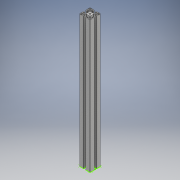
# Autodesk Inventor part: Perfil de Aluminio
Saved by Autodesk Inventor 2018.3 (Build 223284000, 284)
## iProperties
Created: 2020-12-03
Part Number: Perfil de Aluminio
Material: Aluminio 6061
Document SubType Name: Modeling
Designer: SERGIO ROMO
Density: 2.7 g/cm^3
Appearance: Aluminio fundido
Author: SERGIO ROMO
Revision Number: ANY
Autodesk Inventor part; units mm, degrees
ref_plane "YZ Plane" through (0, 0, 0) normal (1, 0, 0) x (0, 1, 0)
ref_plane "XZ Plane" through (0, 0, 0) normal (0, 1, 0) x (-1, 0, 0)
ref_plane "XY Plane" through (0, 0, 0) normal (0, 0, 1) x (1, 0, 0)
sketch "Boceto1" plane through (0, 0, 0) normal (0, 0, 1) x (1, 0, 0)
  line L0 (1.5, 20) -> (15.2768, 20) projected
  line L1 (15.2768, 20) -> (1.5, 20)
  line L2 (8, 12.6183) -> (8, 17.77) projected
  line L3 (8, 17.77) -> (8, 12.6183)
  line L4 (1.5, 12.6183) -> (1.5, 17) projected
  line L5 (2.23, 12) -> (7.3817, 12) projected
  line L6 (7.3817, 18.5) -> (3, 18.5) projected
  line L7 (7.3817, 18.5) -> (3, 18.5)
  arc A0 (3, 18.5) -> (1.9393, 18.0607) centre (3, 17) ccw
  arc A1 (8, 17.77) -> (7.3817, 18.5) centre (7.2949, 17.7996) ccw
  arc A2 (7.8053, 12.1947) -> (8, 12.6183) centre (7.3305, 12.6695) ccw
  line L8 (16, 19.2235) -> (16, 16.1235) projected
  line L9 (16, 19.2235) -> (16, 16.1235)
  circle A3 centre (20, 0) radius 3.4 projected
  arc A4 (1.5, 20) -> (0, 18.5) centre (1.5, 18.5) ccw projected
  arc A5 (1.5, 20) -> (0.4393, 19.5607) centre (1.5, 18.5) ccw
  line L10 (15.4384, 15.5) -> (13.3245, 15.5) projected
  line L11 (15.4384, 15.5) -> (13.3245, 15.5)
  line L12 (13, 15.7733) -> (13, 18.5) projected
  arc A6 (13, 18.5) -> (10, 15.5) centre (13, 15.5) ccw projected
  line L13 (13, 15.7733) -> (13, 18.5)
  line L14 (10, 13.2043) -> (10, 15.5) projected
  line L15 (10, 15.5) -> (10, 13.2043)
  arc A7 (16, 19.2235) -> (15.2768, 20) centre (15.0156, 19.0317) ccw
  arc A8 (15.4384, 15.5) -> (16, 16.1235) centre (15.3104, 16.1799) ccw
  arc A9 (13, 18.5) -> (10, 15.5) centre (13, 15.5) ccw
  line L16 (24, 7.75) -> (16, 7.75) projected
  line L17 (10.8789, 10.9836) -> (13.3701, 8.4924) projected
  line L18 (10.8789, 10.9836) -> (13.3701, 8.4924)
  arc A10 (10, 13.2043) -> (10.8789, 10.9836) centre (13.2448, 13.2043) ccw
  arc A11 (13.3701, 8.4924) -> (16, 7.75) centre (15.5379, 11.1424) ccw
  line L19 (7.3817, 12) -> (7.2793, 12)
  line L20 (2.3351, 12) -> (2.23, 12)
  arc A12 (13, 15.7733) -> (13.3245, 15.5) centre (13.4072, 15.9275) ccw
  line L21 (0, 18.5) -> (0, 4.7232)
  line L22 (7.3817, 12) -> (2.23, 12)
  line L23 (1.5, 12.6183) -> (1.5, 17)
  arc A13 (1.9393, 18.0607) -> (1.5, 17) centre (3, 17) ccw
  arc A14 (1.5, 12.6183) -> (2.23, 12) centre (2.2004, 12.7051) ccw
  arc A15 (7.3817, 12) -> (7.8053, 12.1947) centre (7.3305, 12.6695) ccw
  line L24 (0.7765, 4) -> (3.8765, 4)
  arc A16 (0.4393, 19.5607) -> (0, 18.5) centre (1.5, 18.5) ccw
  line L25 (4.5, 4.5616) -> (4.5, 6.6755)
  line L26 (4.2267, 7) -> (1.5, 7)
  line L27 (4.5, 10) -> (6.7957, 10)
  arc A17 (0, 4.7232) -> (0.7765, 4) centre (0.9683, 4.9844) ccw
  arc A18 (3.8765, 4) -> (4.5, 4.5616) centre (3.8201, 4.6896) ccw
  arc A19 (4.5, 10) -> (1.5, 7) centre (4.5, 7) ccw
  line L28 (12.25, 4) -> (12.25, 0)
  line L29 (9.0164, 9.1211) -> (11.5076, 6.6299)
  arc A20 (9.0164, 9.1211) -> (6.7957, 10) centre (6.7957, 6.7552) ccw
  arc A21 (12.25, 4) -> (11.5076, 6.6299) centre (8.8576, 4.4621) ccw
  arc A22 (4.5, 6.6755) -> (4.2267, 7) centre (4.0725, 6.5928) ccw
  line L30 (1.5, -20) -> (15.2768, -20)
  line L31 (15.2768, -20) -> (1.5, -20)
  line L32 (8, -12.6183) -> (8, -17.77)
  line L33 (8, -17.77) -> (8, -12.6183)
  line L34 (1.5, -12.6183) -> (1.5, -17)
  line L35 (2.23, -12) -> (7.3817, -12)
  line L36 (7.3817, -18.5) -> (3, -18.5)
  line L37 (7.3817, -18.5) -> (3, -18.5)
  arc A23 (1.9393, -18.0607) -> (3, -18.5) centre (3, -17) ccw
  arc A24 (7.3817, -18.5) -> (8, -17.77) centre (7.2949, -17.7996) ccw
  arc A25 (8, -12.6183) -> (7.8053, -12.1947) centre (7.3305, -12.6695) ccw
  line L38 (16, -19.2235) -> (16, -16.1235)
  arc A26 (0, -18.5) -> (1.5, -20) centre (1.5, -18.5) ccw
  arc A27 (0.4393, -19.5607) -> (1.5, -20) centre (1.5, -18.5) ccw
  line L39 (15.4384, -15.5) -> (13.3245, -15.5)
  line L40 (13, -15.7733) -> (13, -18.5)
  arc A28 (10, -15.5) -> (13, -18.5) centre (13, -15.5) ccw
  line L41 (13, -15.7733) -> (13, -18.5)
  line L42 (10, -13.2043) -> (10, -15.5)
  line L43 (10, -15.5) -> (10, -13.2043)
  arc A29 (15.2768, -20) -> (16, -19.2235) centre (15.0156, -19.0317) ccw
  arc A30 (16, -16.1235) -> (15.4384, -15.5) centre (15.3104, -16.1799) ccw
  arc A31 (10, -15.5) -> (13, -18.5) centre (13, -15.5) ccw
  line L44 (24, -7.75) -> (16, -7.75)
  line L45 (10.8789, -10.9836) -> (13.3701, -8.4924)
  line L46 (10.8789, -10.9836) -> (13.3701, -8.4924)
  arc A32 (10.8789, -10.9836) -> (10, -13.2043) centre (13.2448, -13.2043) ccw
  arc A33 (16, -7.75) -> (13.3701, -8.4924) centre (15.5379, -11.1424) ccw
  line L47 (7.3817, -12) -> (7.2793, -12)
  line L48 (2.3351, -12) -> (2.23, -12)
  arc A34 (13.3245, -15.5) -> (13, -15.7733) centre (13.4072, -15.9275) ccw
  arc A35 (0, -18.5) -> (0.4393, -19.5607) centre (1.5, -18.5) ccw
  line L49 (0, -18.5) -> (0, -4.7232)
  arc A36 (0.7765, -4) -> (0, -4.7232) centre (0.9683, -4.9844) ccw
  line L50 (0.7765, -4) -> (3.8765, -4)
  arc A37 (4.5, -4.5616) -> (3.8765, -4) centre (3.8201, -4.6896) ccw
  line L51 (4.5, -4.5616) -> (4.5, -6.6755)
  arc A38 (4.2267, -7) -> (4.5, -6.6755) centre (4.0725, -6.5928) ccw
  line L52 (4.2267, -7) -> (1.5, -7)
  arc A39 (1.5, -7) -> (4.5, -10) centre (4.5, -7) ccw
  line L53 (4.5, -10) -> (6.7957, -10)
  arc A40 (6.7957, -10) -> (9.0164, -9.1211) centre (6.7957, -6.7552) ccw
  line L54 (9.0164, -9.1211) -> (11.5076, -6.6299)
  arc A41 (11.5076, -6.6299) -> (12.25, -4) centre (8.8576, -4.4621) ccw
  line L55 (12.25, -4) -> (12.25, 0)
  arc A42 (7.8053, -12.1947) -> (7.3817, -12) centre (7.3305, -12.6695) ccw
  line L56 (7.3817, -12) -> (2.23, -12)
  arc A43 (2.23, -12) -> (1.5, -12.6183) centre (2.2004, -12.7051) ccw
  line L57 (1.5, -12.6183) -> (1.5, -17)
  arc A44 (1.5, -17) -> (1.9393, -18.0607) centre (3, -17) ccw
  line L58 (38.5, 20) -> (24.7232, 20)
  line L59 (24.7232, 20) -> (38.5, 20)
  line L60 (32, 12.6183) -> (32, 17.77)
  line L61 (32, 17.77) -> (32, 12.6183)
  line L62 (38.5, 12.6183) -> (38.5, 17)
  line L63 (37.77, 12) -> (32.6183, 12)
  line L64 (32.6183, 18.5) -> (37, 18.5)
  line L65 (32.6183, 18.5) -> (37, 18.5)
  arc A45 (38.0607, 18.0607) -> (37, 18.5) centre (37, 17) ccw
  arc A46 (32.6183, 18.5) -> (32, 17.77) centre (32.7051, 17.7996) ccw
  arc A47 (32, 12.6183) -> (32.1947, 12.1947) centre (32.6695, 12.6695) ccw
  line L66 (24, 19.2235) -> (24, 16.1235)
  line L67 (24, 19.2235) -> (24, 16.1235)
  arc A48 (40, 18.5) -> (38.5, 20) centre (38.5, 18.5) ccw
  arc A49 (39.5607, 19.5607) -> (38.5, 20) centre (38.5, 18.5) ccw
  line L68 (24.5616, 15.5) -> (26.6755, 15.5)
  line L69 (24.5616, 15.5) -> (26.6755, 15.5)
  line L70 (27, 15.7733) -> (27, 18.5)
  arc A50 (30, 15.5) -> (27, 18.5) centre (27, 15.5) ccw
  line L71 (27, 15.7733) -> (27, 18.5)
  line L72 (30, 13.2043) -> (30, 15.5)
  line L73 (30, 15.5) -> (30, 13.2043)
  arc A51 (24.7232, 20) -> (24, 19.2235) centre (24.9844, 19.0317) ccw
  arc A52 (24, 16.1235) -> (24.5616, 15.5) centre (24.6896, 16.1799) ccw
  arc A53 (30, 15.5) -> (27, 18.5) centre (27, 15.5) ccw
  line L74 (29.1211, 10.9836) -> (26.6299, 8.4924)
  line L75 (29.1211, 10.9836) -> (26.6299, 8.4924)
  arc A54 (29.1211, 10.9836) -> (30, 13.2043) centre (26.7552, 13.2043) ccw
  arc A55 (24, 7.75) -> (26.6299, 8.4924) centre (24.4621, 11.1424) ccw
  line L76 (32.6183, 12) -> (32.7207, 12)
  line L77 (37.6649, 12) -> (37.77, 12)
  arc A56 (26.6755, 15.5) -> (27, 15.7733) centre (26.5928, 15.9275) ccw
  arc A57 (40, 18.5) -> (39.5607, 19.5607) centre (38.5, 18.5) ccw
  line L78 (40, 18.5) -> (40, 4.7232)
  arc A58 (39.2235, 4) -> (40, 4.7232) centre (39.0317, 4.9844) ccw
  line L79 (39.2235, 4) -> (36.1235, 4)
  arc A59 (35.5, 4.5616) -> (36.1235, 4) centre (36.1799, 4.6896) ccw
  line L80 (35.5, 4.5616) -> (35.5, 6.6755)
  arc A60 (35.7733, 7) -> (35.5, 6.6755) centre (35.9275, 6.5928) ccw
  line L81 (35.7733, 7) -> (38.5, 7)
  arc A61 (38.5, 7) -> (35.5, 10) centre (35.5, 7) ccw
  line L82 (35.5, 10) -> (33.2043, 10)
  arc A62 (33.2043, 10) -> (30.9836, 9.1211) centre (33.2043, 6.7552) ccw
  line L83 (30.9836, 9.1211) -> (28.4924, 6.6299)
  arc A63 (28.4924, 6.6299) -> (27.75, 4) centre (31.1424, 4.4621) ccw
  line L84 (27.75, 4) -> (27.75, 0)
  arc A64 (32.1947, 12.1947) -> (32.6183, 12) centre (32.6695, 12.6695) ccw
  line L85 (32.6183, 12) -> (37.77, 12)
  arc A65 (37.77, 12) -> (38.5, 12.6183) centre (37.7996, 12.7051) ccw
  line L86 (38.5, 12.6183) -> (38.5, 17)
  arc A66 (38.5, 17) -> (38.0607, 18.0607) centre (37, 17) ccw
  arc A67 (38.0607, -18.0607) -> (38.5, -17) centre (37, -17) ccw
  arc A68 (37, -18.5) -> (38.0607, -18.0607) centre (37, -17) ccw
  arc A69 (38.5, -20) -> (39.5607, -19.5607) centre (38.5, -18.5) ccw
  arc A70 (39.5607, -19.5607) -> (40, -18.5) centre (38.5, -18.5) ccw
  arc A71 (38.5, -20) -> (40, -18.5) centre (38.5, -18.5) ccw
  line L87 (30, -13.2043) -> (30, -15.5)
  line L88 (29.1211, -10.9836) -> (26.6299, -8.4924)
  line L89 (29.1211, -10.9836) -> (26.6299, -8.4924)
  arc A72 (30, -13.2043) -> (29.1211, -10.9836) centre (26.7552, -13.2043) ccw
  line L90 (30, -15.5) -> (30, -13.2043)
  line L91 (38.5, -20) -> (24.7232, -20)
  line L92 (24.7232, -20) -> (38.5, -20)
  arc A73 (27, -15.7733) -> (26.6755, -15.5) centre (26.5928, -15.9275) ccw
  arc A74 (27, -18.5) -> (30, -15.5) centre (27, -15.5) ccw
  arc A75 (27, -18.5) -> (30, -15.5) centre (27, -15.5) ccw
  line L93 (27, -15.7733) -> (27, -18.5)
  line L94 (27, -15.7733) -> (27, -18.5)
  line L95 (27.75, -4) -> (27.75, 0)
  arc A76 (27.75, -4) -> (28.4924, -6.6299) centre (31.1424, -4.4621) ccw
  line L96 (30.9836, -9.1211) -> (28.4924, -6.6299)
  arc A77 (30.9836, -9.1211) -> (33.2043, -10) centre (33.2043, -6.7552) ccw
  arc A78 (36.1235, -4) -> (35.5, -4.5616) centre (36.1799, -4.6896) ccw
  line L97 (35.5, -4.5616) -> (35.5, -6.6755)
  arc A79 (35.5, -6.6755) -> (35.7733, -7) centre (35.9275, -6.5928) ccw
  line L98 (35.5, -10) -> (33.2043, -10)
  line L99 (39.2235, -4) -> (36.1235, -4)
  arc A80 (40, -4.7232) -> (39.2235, -4) centre (39.0317, -4.9844) ccw
  line L100 (35.7733, -7) -> (38.5, -7)
  arc A81 (35.5, -10) -> (38.5, -7) centre (35.5, -7) ccw
  line L101 (32, -12.6183) -> (32, -17.77)
  line L102 (32, -17.77) -> (32, -12.6183)
  line L103 (32.6183, -18.5) -> (37, -18.5)
  line L104 (32.6183, -18.5) -> (37, -18.5)
  arc A82 (32, -17.77) -> (32.6183, -18.5) centre (32.7051, -17.7996) ccw
  line L105 (40, -18.5) -> (40, -4.7232)
  line L106 (38.5, -12.6183) -> (38.5, -17)
  line L107 (38.5, -12.6183) -> (38.5, -17)
  arc A83 (38.5, -12.6183) -> (37.77, -12) centre (37.7996, -12.7051) ccw
  line L108 (37.6649, -12) -> (37.77, -12)
  line L109 (32.6183, -12) -> (37.77, -12)
  line L110 (37.77, -12) -> (32.6183, -12)
  line L111 (32.6183, -12) -> (32.7207, -12)
  arc A84 (32.6183, -12) -> (32.1947, -12.1947) centre (32.6695, -12.6695) ccw
  arc A85 (32.1947, -12.1947) -> (32, -12.6183) centre (32.6695, -12.6695) ccw
  arc A86 (24, -19.2235) -> (24.7232, -20) centre (24.9844, -19.0317) ccw
  line L112 (24, -19.2235) -> (24, -16.1235)
  arc A87 (24.5616, -15.5) -> (24, -16.1235) centre (24.6896, -16.1799) ccw
  line L113 (24.5616, -15.5) -> (26.6755, -15.5)
  arc A88 (26.6299, -8.4924) -> (24, -7.75) centre (24.4621, -11.1424) ccw
  line L114 (16, 7.75) -> (24, 7.75)
  point P0 (0, 0)
  point P1 (40, 0)
  constraints: 208 end point, 176 point on circle, 86 centre point, 5 collinear, 3 horizontal, 3 vertical, 2 tangent
extrude "Extrusión1" add sketch "Boceto1" along normal blind 500
